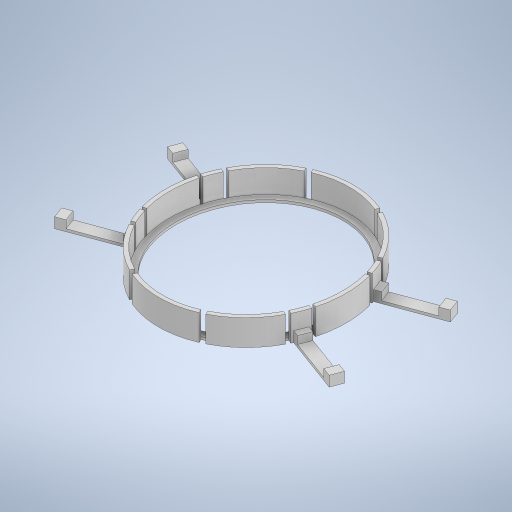
# Autodesk Inventor part: calibracao(0,5cm)
Saved by Autodesk Inventor 2024.3 (Build 283343000, 343)
## iProperties
Created: 2024-12-11
Part Number: calibracao(0,5cm)
Material: Genérico
Document SubType Name: Modeling
Designer: lostv
Density: 1 g/cm^3
Appearance: Padrão
Author: lostv
Autodesk Inventor part; units mm, degrees
ref_plane "YZ Plane" through (0, 0, 0) normal (1, 0, 0) x (0, 1, 0)
ref_plane "XZ Plane" through (0, 0, 0) normal (0, 1, 0) x (-1, 0, 0)
ref_plane "XY Plane" through (0, 0, 0) normal (0, 0, 1) x (1, 0, 0)
sketch "Esboço1" plane through (0, 0, 0) normal (0, 1, 0) x (-1, 0, 0)
  ellipse E0 centre (-16.8231, 43.9447) end of major axis (58.1769, 43.9447) minor radius 80.5 (58.1769, 43.9447) -> (-16.8231, 124.4447) ccw
  line L0 (-16.8231, 124.4447) -> (-16.8231, 43.9447) construction
  line L1 (-16.8231, 43.9447) -> (58.1769, 43.9447)
  line L2 (-16.8231, 43.9447) -> (38.0514, 98.8191) construction
  line L3 (-16.8231, 43.9447) -> (60.7811, 43.9447) construction
  line L4 (58.1769, 43.9447) -> (61.1769, 43.9447)
  ellipse E1 centre (-16.8231, 43.9447) end of major axis (-16.8231, 127.4447) minor radius 78 (36.942, 104.4388) -> (-11.8231, 127.273) ccw
  ellipse E2 centre (-16.8231, 43.9447) end of major axis (-16.8231, 127.4447) minor radius 78 (61.0369, 48.9447) -> (43.4965, 96.8842) ccw
  ellipse E3 centre (-16.8231, 43.9447) end of major axis (-16.8231, 127.4447) minor radius 78 (-21.8231, 127.273) -> (-70.5882, 104.4388) ccw
  ellipse E4 centre (-16.8231, 43.9447) end of major axis (-91.8231, 43.9447) minor radius 80.5 (-16.8231, 124.4447) -> (-91.8231, 43.9447) ccw
  line L5 (-16.8231, 43.9447) -> (-71.6976, 98.8191) construction
  line L6 (-16.8231, 43.9447) -> (-91.8231, 43.9447) construction
  line L7 (-16.8231, 43.9447) -> (-91.8231, 43.9447)
  ellipse E5 centre (-16.8231, 43.9447) end of major axis (-16.8231, 127.4447) minor radius 78 (-77.1427, 96.8842) -> (-94.6831, 48.9447) ccw
  line L8 (-96.047, 46.9447) -> (-91.771, 46.9447)
  line L9 (58.1769, 43.9447) -> (-91.8231, 43.9447)
  line L10 (-16.8231, 43.9447) -> (38.0514, -10.9298) construction
  ellipse E6 centre (-16.8231, 43.9447) end of major axis (58.1769, 43.9447) minor radius 80.5 (-16.8231, -36.5553) -> (58.1769, 43.9447) ccw
  line L11 (-16.8231, -36.5553) -> (-16.8231, 43.9447) construction
  line L12 (-13.8231, -40.7731) -> (-13.8231, -36.4909)
  line L13 (-11.8231, -40.7731) -> (-11.8231, -36.3762)
  line L14 (-13.8231, -36.4909) -> (-13.8231, -40.7731)
  ellipse E7 centre (-16.8231, 43.9447) end of major axis (-16.8231, -39.5553) minor radius 78 (-11.8231, -39.3836) -> (36.942, -16.5494) ccw
  ellipse E8 centre (-16.8231, 43.9447) end of major axis (-16.8231, -39.5553) minor radius 78 (43.4965, -8.9948) -> (61.0369, 38.9447) ccw
  line L15 (-69.7437, -13.0978) -> (-72.9021, -15.9416)
  line L16 (-73.673, -8.5619) -> (-76.9169, -11.4827)
  line L17 (-73.673, -8.5619) -> (-76.9169, -11.4827)
  line L18 (-69.7437, -13.0978) -> (-72.9021, -15.9416)
  line L19 (-19.8231, -40.7731) -> (-19.8231, -36.4909)
  line L20 (-19.8231, -36.4909) -> (-19.8231, -40.7731)
  line L21 (-21.8231, -40.7731) -> (-21.8231, -36.3762)
  ellipse E9 centre (-16.8231, 43.9447) end of major axis (-16.8231, -39.5553) minor radius 78 (-70.5882, -16.5494) -> (-21.8231, -39.3836) ccw
  line L22 (-16.8231, 43.9447) -> (-71.6976, -10.9298) construction
  ellipse E10 centre (-16.8231, 43.9447) end of major axis (-91.8231, 43.9447) minor radius 80.5 (-91.8231, 43.9447) -> (-16.8231, -36.5553) ccw
  ellipse E11 centre (-16.8231, 43.9447) end of major axis (-16.8231, -39.5553) minor radius 78 (-94.6831, 38.9447) -> (-77.1427, -8.9948) ccw
  line L23 (-96.047, 40.9447) -> (-91.8, 40.9447)
  line L24 (23.1769, -78.0731) -> (-56.8231, -78.0731)
  line L25 (-56.8231, -78.0731) -> (-56.8231, -78.0731)
  line L26 (-16.8231, -78.0731) -> (-16.8231, -84.5751) construction
  line L27 (-96.047, 38.9447) -> (-91.6783, 38.9447)
  line L28 (-96.047, 48.9447) -> (-91.6783, 48.9447)
  line L29 (-96.047, 38.9447) -> (-98.347, 38.9447) construction
  line L30 (-98.347, 38.9447) -> (-98.347, 41.4447) construction
  line L31 (-98.347, 41.4447) -> (-96.047, 41.4447) construction
  line L32 (-96.047, 38.9447) -> (-98.347, 38.9447)
  line L33 (-98.347, 41.4447) -> (-98.347, 38.9447)
  line L34 (-98.347, 41.4447) -> (-96.047, 41.4447)
  line L35 (-96.047, 41.4447) -> (-96.047, 40.9447)
  line L36 (-96.047, 46.9447) -> (-96.047, 46.4447)
  line L37 (-98.347, 46.4447) -> (-96.047, 46.4447)
  line L38 (-98.347, 46.4447) -> (-98.347, 48.9447)
  line L39 (-98.347, 48.9447) -> (-96.047, 48.9447)
  line L40 (-96.047, 40.9447) -> (-96.047, 41.4447) construction
  line L41 (-96.047, 46.4447) -> (-96.047, 46.9447) construction
  line L42 (-96.047, 41.4447) -> (-96.047, 46.4447)
  line L43 (-72.9021, -15.9416) -> (-76.9169, -11.4827) construction
  line L44 (-78.2551, -9.9964) -> (-74.9072, -6.9819)
  line L45 (-71.5638, -17.4279) -> (-68.3579, -14.5413)
  line L46 (-71.5638, -17.4279) -> (-73.2731, -18.9669)
  line L47 (-73.2731, -18.9669) -> (-74.9459, -17.109)
  line L48 (-74.9459, -17.109) -> (-73.2367, -15.57)
  line L49 (-72.9021, -15.9416) -> (-73.2367, -15.57)
  line L50 (-76.9169, -11.4827) -> (-73.2367, -15.57)
  line L51 (-78.2551, -9.9964) -> (-79.9644, -11.5354)
  line L52 (-79.9644, -11.5354) -> (-78.2915, -13.3933)
  line L53 (-78.2915, -13.3933) -> (-76.5823, -11.8543)
  line L54 (-13.8231, -40.7731) -> (-19.8231, -40.7731) construction
  line L55 (-21.8231, -40.7731) -> (-21.8231, -43.0731)
  line L56 (-21.8231, -43.0731) -> (-19.3231, -43.0731)
  line L57 (-19.3231, -43.0731) -> (-19.3231, -40.7731)
  line L58 (-19.8231, -40.7731) -> (-19.3231, -40.7731)
  line L59 (-11.8231, -40.7731) -> (-11.8231, -43.0731)
  line L60 (-11.8231, -43.0731) -> (-14.3231, -43.0731)
  line L61 (-14.3231, -43.0731) -> (-14.3231, -40.7731)
  line L62 (-13.8231, -40.7731) -> (-14.3231, -40.7731)
  line L63 (-19.3231, -40.7731) -> (-14.3231, -40.7731)
  line L64 (46.3182, -11.5354) -> (44.6453, -13.3933)
  line L65 (44.6089, -9.9964) -> (46.3182, -11.5354)
  line L66 (44.6453, -13.3933) -> (42.9361, -11.8543)
  line L67 (40.0268, -8.5619) -> (43.2707, -11.4827)
  line L68 (44.6089, -9.9964) -> (41.261, -6.9819)
  line L69 (43.2707, -11.4827) -> (39.5905, -15.57)
  line L70 (39.2559, -15.9416) -> (43.2707, -11.4827) construction
  line L71 (36.0975, -13.0978) -> (39.2559, -15.9416)
  line L72 (39.2559, -15.9416) -> (39.5905, -15.57)
  line L73 (41.2997, -17.109) -> (39.5905, -15.57)
  line L74 (39.6269, -18.9669) -> (41.2997, -17.109)
  line L75 (37.9176, -17.4279) -> (39.6269, -18.9669)
  line L76 (37.9176, -17.4279) -> (34.7117, -14.5413)
  line L77 (62.4009, 38.9447) -> (64.7009, 38.9447)
  line L78 (64.7009, 38.9447) -> (64.7009, 41.4447)
  line L79 (64.7009, 41.4447) -> (62.4009, 41.4447)
  line L80 (62.4009, 41.4447) -> (62.4009, 40.9447)
  line L81 (62.4009, 40.9447) -> (58.1538, 40.9447)
  line L82 (62.4009, 38.9447) -> (58.0321, 38.9447)
  line L83 (62.4009, 41.4447) -> (62.4009, 46.4447)
  line L84 (64.7009, 46.4447) -> (62.4009, 46.4447)
  line L85 (62.4009, 46.9447) -> (62.4009, 46.4447)
  line L86 (64.7009, 46.4447) -> (64.7009, 48.9447)
  line L87 (64.7009, 48.9447) -> (62.4009, 48.9447)
  line L88 (62.4009, 48.9447) -> (58.0321, 48.9447)
  line L89 (62.4009, 46.9447) -> (58.1248, 46.9447)
  line L90 (39.2559, 103.831) -> (39.5905, 103.4594)
  line L91 (37.9176, 105.3172) -> (39.6269, 106.8562)
  line L92 (39.6269, 106.8562) -> (41.2997, 104.9984)
  line L93 (41.2997, 104.9984) -> (39.5905, 103.4594)
  line L94 (39.2559, 103.831) -> (43.2707, 99.3721) construction
  line L95 (43.2707, 99.3721) -> (39.5905, 103.4594)
  line L96 (44.6453, 101.2827) -> (42.9361, 99.7437)
  line L97 (46.3182, 99.4248) -> (44.6453, 101.2827)
  line L98 (44.6089, 97.8858) -> (46.3182, 99.4248)
  line L99 (44.6089, 97.8858) -> (41.261, 94.8713)
  line L100 (40.0268, 96.4513) -> (43.2707, 99.3721)
  line L101 (36.0975, 100.9871) -> (39.2559, 103.831)
  line L102 (37.9176, 105.3172) -> (34.7117, 102.4306)
  line L103 (-71.5638, 105.3172) -> (-68.3579, 102.4306)
  line L104 (-71.5638, 105.3172) -> (-73.2731, 106.8562)
  line L105 (-73.2731, 106.8562) -> (-74.9459, 104.9984)
  line L106 (-74.9459, 104.9984) -> (-73.2367, 103.4594)
  line L107 (-72.9021, 103.831) -> (-73.2367, 103.4594)
  line L108 (-69.7437, 100.9871) -> (-72.9021, 103.831)
  line L109 (-76.9169, 99.3721) -> (-73.2367, 103.4594)
  line L110 (-78.2915, 101.2827) -> (-76.5823, 99.7437)
  line L111 (-73.673, 96.4513) -> (-76.9169, 99.3721)
  line L112 (-79.9644, 99.4248) -> (-78.2915, 101.2827)
  line L113 (-78.2551, 97.8858) -> (-79.9644, 99.4248)
  line L114 (-78.2551, 97.8858) -> (-74.9072, 94.8713)
  line L115 (-21.8231, 128.6625) -> (-21.8231, 130.9625)
  line L116 (-21.8231, 128.6625) -> (-21.8231, 124.2656)
  line L117 (-21.8231, 130.9625) -> (-19.3231, 130.9625)
  line L118 (-19.3231, 130.9625) -> (-19.3231, 128.6625)
  line L119 (-19.8231, 128.6625) -> (-19.3231, 128.6625)
  line L120 (-19.8231, 128.6625) -> (-19.8231, 124.3803)
  line L121 (-19.3231, 128.6625) -> (-14.3231, 128.6625)
  line L122 (-14.3231, 130.9625) -> (-14.3231, 128.6625)
  line L123 (-11.8231, 130.9625) -> (-14.3231, 130.9625)
  line L124 (-11.8231, 128.6625) -> (-11.8231, 124.2656)
  line L125 (-11.8231, 128.6625) -> (-11.8231, 130.9625)
  line L126 (-13.8231, 128.6625) -> (-13.8231, 124.3803)
  line L127 (-13.8231, 128.6625) -> (-19.8231, 128.6625) construction
  line L128 (-13.8231, 128.6625) -> (-14.3231, 128.6625)
  line L129 (58.1538, 40.9447) -> (58.1248, 40.9447)
  line L130 (-91.8, 40.9447) -> (-91.771, 40.9447)
  line L131 (-56.8231, -78.0731) -> (23.1769, -78.0731)
  line L132 (23.1769, -78.0731) -> (23.1769, -43.0731)
  line L133 (-56.8231, -43.0731) -> (-56.8231, -78.0731)
  line L134 (-16.8231, 43.9447) -> (-16.8231, 155.9447) construction
  line L135 (-16.8231, 43.9447) -> (89.6769, 43.9447) construction
  line L136 (-16.8231, 43.9447) -> (-16.8231, -64.5553) construction
  line L137 (-16.8231, 43.9447) -> (-123.3231, 43.9447) construction
  line L138 (-16.8231, 43.9447) -> (92.6769, 43.9447) construction
  line L139 (-16.8231, 43.9447) -> (-126.3231, 43.9447) construction
  line L140 (-16.8231, 43.9447) -> (-16.8231, 158.9447) construction
  line L141 (-16.8231, 43.9447) -> (-16.8231, -67.5553) construction
  line L142 (-14.3231, -43.0731) -> (-14.3231, -40.7731)
  line L143 (-19.3231, -40.7731) -> (-19.3231, -43.0731)
  line L144 (-19.3231, -40.7731) -> (-14.3231, -40.7731)
  line L145 (23.1769, -43.0731) -> (-14.3231, -43.0731)
  line L146 (-19.3231, -43.0731) -> (-56.8231, -43.0731)
  ellipse E12 centre (-16.8231, 43.9447) end of major axis (92.6769, 43.9447) minor radius 115 (23.1769, -63.1078) -> (-56.8231, -63.1078) ccw
  line L147 (81.5648, 71.8126) -> (78.4536, 83.201)
  line L148 (78.4536, 83.201) -> (82.5191, 84.3116)
  line L149 (81.5648, 71.8126) -> (86.023, 73.0305)
  line L150 (-115.211, 71.8126) -> (-119.6692, 73.0305)
  line L151 (-115.211, 71.8126) -> (-112.0998, 83.201)
  line L152 (-112.0998, 83.201) -> (-116.1653, 84.3116)
  ellipse E13 centre (-16.8231, 43.9447) end of major axis (89.6769, 43.9447) minor radius 112 (23.1769, -59.8555) -> (86.023, 73.0305) ccw
  ellipse E14 centre (-16.8231, 43.9447) end of major axis (89.6769, 43.9447) minor radius 112 (82.5191, 84.3116) -> (-116.1653, 84.3116) ccw
  ellipse E15 centre (-16.8231, 43.9447) end of major axis (89.6769, 43.9447) minor radius 112 (-119.6692, 73.0305) -> (-56.8231, -59.8555) ccw
  circle A0 centre (16.1769, -50.0731) radius 1.75
  circle A1 centre (-49.8231, -50.0731) radius 1.75
  line L153 (89.5899, 93.6335) -> (44.298, 76.9085)
  line L154 (44.298, 76.9085) -> (47.1282, 68.1314)
  line L155 (47.1282, 68.1314) -> (92.7817, 84.99)
  line L156 (92.7817, 84.99) -> (89.5899, 93.6335)
  line L157 (89.5899, -5.7442) -> (44.298, 10.9809)
  line L158 (44.298, 10.9809) -> (47.1282, 19.758)
  line L159 (47.1282, 19.758) -> (92.7817, 2.8994)
  line L160 (92.7817, 2.8994) -> (89.5899, -5.7442)
  line L161 (-123.2361, 93.6335) -> (-77.9442, 76.9085)
  line L162 (-77.9442, 76.9085) -> (-80.7744, 68.1314)
  line L163 (-80.7744, 68.1314) -> (-126.4279, 84.99)
  line L164 (-126.4279, 84.99) -> (-123.2361, 93.6335)
  line L165 (-123.2361, -5.7442) -> (-77.9442, 10.9809)
  line L166 (-80.7744, 19.758) -> (-126.4279, 2.8994)
  line L167 (-126.4279, 2.8994) -> (-123.2361, -5.7442)
  line L168 (-77.9442, 10.9809) -> (-80.7744, 19.758)
  line L169 (-16.8231, 43.9447) -> (-16.8231, -31.5553) construction
  line L170 (-16.8231, 43.9447) -> (53.1769, 43.9447) construction
  ellipse E16 centre (-16.8231, 43.9447) end of major axis (-16.8231, -31.5553) minor radius 70
  line L171 (-16.8231, 43.9447) -> (-16.8231, -28.5553) construction
  line L172 (-16.8231, 43.9447) -> (50.1769, 43.9447) construction
  ellipse E17 centre (-16.8231, 43.9447) end of major axis (-16.8231, -28.5553) minor radius 67
  line L173 (9.1801, 114.0421) -> (7.9104, 111.3238)
  line L174 (12.7897, 112.3561) -> (11.5281, 109.634)
  line L175 (9.1801, -26.1528) -> (7.9104, -23.4345)
  line L176 (12.7897, -24.4667) -> (11.5281, -21.7446)
  line L177 (-42.8263, 114.0421) -> (-41.5566, 111.3238)
  line L178 (-46.4359, 112.3561) -> (-45.1743, 109.634)
  line L179 (-42.8263, -26.1528) -> (-41.5566, -23.4345)
  line L180 (-46.4359, -24.4667) -> (-45.1743, -21.7446)
  line L181 (-77.4369, 81.7095) -> (-74.7161, 80.4386)
  line L182 (-76.0765, 77.7854) -> (-78.8404, 78.9584)
  line L183 (-80.4928, 66.5177) -> (-83.3871, 67.3084)
  line L184 (-81.1396, 64.2577) -> (-84.0231, 65.0848)
  line L185 (43.7907, 81.7095) -> (41.0699, 80.4386)
  line L186 (42.4303, 77.7854) -> (45.1942, 78.9584)
  line L187 (46.8466, 66.5177) -> (49.7409, 67.3084)
  line L188 (47.4934, 64.2577) -> (50.3769, 65.0848)
  line L189 (-77.4369, 6.1798) -> (-74.7161, 7.4508)
  line L190 (-76.0765, 10.1039) -> (-78.8404, 8.931)
  line L191 (-80.4928, 21.3717) -> (-83.3871, 20.581)
  line L192 (-81.1396, 23.6316) -> (-84.0231, 22.8046)
  line L193 (47.4934, 23.6316) -> (50.3769, 22.8046)
  line L194 (46.8466, 21.3717) -> (49.7409, 20.581)
  line L195 (42.4303, 10.1039) -> (45.1942, 8.931)
  line L196 (43.7907, 6.1798) -> (41.0699, 7.4508)
  line L197 (-16.8231, 43.9447) -> (45.1769, 43.9447)
  line L198 (-16.8231, 43.9447) -> (-16.8231, -23.5553)
  ellipse E18 centre (-16.8231, 43.9447) end of major axis (45.1769, 43.9447) minor radius 67.5
  point P0 (0, 0)
  point P1 (78.1769, 43.9447)
  point P2 (81.1769, 43.9447)
  point P3 (-100.7855, 43.9447)
  point P4 (-72.3567, -15.4505)
  point P5 (-97.197, 41.4447)
  point P6 (-97.197, 38.9447)
  point P7 (-96.047, 41.1947)
  point P8 (-96.047, 46.6947)
  point P9 (-97.197, 48.9447)
  point P10 (-93.8627, 48.9447)
  point P11 (-72.4185, -18.1974)
  point P12 (-77.4369, -12.6238)
  point P13 (-79.128, -12.4643)
  point P14 (-14.3231, -41.9231)
  point P15 (-19.5731, -40.7731)
  point P16 (-13.8231, -38.632)
  point P17 (62.4009, 41.1947)
  point P18 (-96.047, 43.9447)
  point P19 (-58.2564, -59.4853)
  point P20 (24.6102, -59.4853)
  point P21 (23.1769, -57.0582)
  point P22 (-13.0731, 130.9625)
  point P23 (64.7009, 40.1947)
  point P24 (-82.8852, 68.9108)
  point P25 (-79.532, 77.4948)
  point P26 (-84.2338, 79.231)
  point P27 (-87.5779, 70.6437)
  point P28 (-79.532, 10.3946)
  point P29 (-82.8852, 18.9785)
  point P30 (-87.5779, 17.2456)
  point P31 (-84.2338, 8.6583)
  point P32 (-119.9522, 82.5987)
  point P33 (-116.6506, 91.2017)
  point P34 (-116.6506, -3.3123)
  point P35 (-119.9522, 5.2907)
  point P36 (83.0044, 91.2017)
  point P37 (86.306, 82.5987)
  point P38 (45.8858, 77.4948)
  point P39 (49.239, 68.9108)
  point P40 (53.9317, 70.6437)
  point P41 (50.5876, 79.231)
  point P42 (86.306, 5.2907)
  point P43 (83.0044, -3.3123)
  point P44 (49.239, 18.9785)
  point P45 (45.8858, 10.3946)
  point P46 (50.5876, 8.6583)
  point P47 (53.9317, 17.2456)
  dimension "d3" = 83.5
  dimension "d4" = 78
  dimension "d0" = 75
  dimension "d1" = 80.5
  dimension "d2" = 45
  dimension "d5" = 2.5
  dimension "d6" = 2
  dimension "d7" = 2.3
  dimension "d8" = 2.3
  dimension "d9" = 2
  dimension "d10" = 2.5
  dimension "d11" = 6.6688
  dimension "d12" = 2.5
  dimension "d13" = 2.5
  dimension "d14" = 2.3
  dimension "d15" = 2.5
  dimension "d16" = 2.5
  dimension "d17" = 2.3
  dimension "d18" = 4.2822
  dimension "d19" = 6
  dimension "d20" = 112
  dimension "d21" = 106.5
  dimension "d22" = 106.5
  dimension "d23" = 109.5
  dimension "d24" = 109.5
  dimension "d25" = 115
  dimension "d26" = 24.9822
  dimension "d27" = 24.9761
  dimension "d28" = 80
  dimension "d29" = 40
  dimension "d30" = 35
  dimension "d31" = 3.5
  dimension "d32" = 7
  dimension "d33" = 7
  dimension "d34" = 75.5
  dimension "d35" = 70
  dimension "d36" = 72.5
  dimension "d37" = 67
  dimension "d46" = 62
  dimension "d47" = 67.5
  constraints: 398 end point, 148 symmetric about line, 55 point on line, 22 perpendicular, 18 coincident, 18 horizontal, 16 midpoint, 14 vertical, 12 collinear, 5 parallel, 2 centre point, 1 equal length, 129 other
  measures "d0" distance of L1.start L1.end
  measures "d1" distance of L0.start L1.start
  measures "d2" angle of L3 L2
  measures "d5" distance of point (-97.197, 41.445) point (-97.197, 38.945)
  measures "d6" distance between parallel lines of L27 L23
  measures "d7" distance from line of point (-96.047, 41.195) L33
  measures "d8" distance from line of point (-96.047, 46.695) L38
  measures "d9" distance from line of L8 point (-93.863, 48.945)
  measures "d10" distance from line of point (-97.197, 48.945) L37
  measures "d11" distance of L27.end L29.end
  measures "d12" distance from line of point (-72.418, -18.197) L48
  measures "d13" distance from line of point (-77.437, -12.624) L51
  measures "d14" distance between parallel lines of L43 L52
  measures "d15" distance between parallel lines of L57 L55
  measures "d16" distance from line of L59 point (-14.323, -41.923)
  measures "d17" distance from line of point (-19.573, -40.773) L56
  measures "d18" distance of L58.start L20.start
  measures "d19" distance from line of point (-13.823, -38.632) L19
  measures "d20" distance of L135.start L134.end
  measures "d21" distance of L135.start L135.end
  measures "d22" distance of L135.start L137.end
  measures "d23" distance of L138.start L138.end
  measures "d24" distance of L138.start L139.end
  measures "d25" distance of L138.start L140.end
  measures "d26" vertical distance of point (-13.073, 130.962) L134.end
  measures "d27" horizontal distance of point (64.701, 40.195) L135.end
  measures "d28" distance between parallel lines of L132 L133
  measures "d29" distance between parallel lines of L136 L132
  measures "d30" distance of L133.start L25.end
  measures "d31" diameter of A0
  measures "d32" distance from line of L132 A0.centre
  measures "d33" distance from line of L145 A0.centre
  measures "d34" distance of L169.start L169.end
  measures "d35" distance of L169.start L170.end
  measures "d36" distance of L171.start L171.end
  measures "d37" distance of L171.start L172.end
  measures "d46" distance of L197.start L197.end
  measures "d47" distance of L198.start L198.end
extrude "Extrusão1" add sketch "Esboço1" along normal blind 2 contours E17 L7 E18 L1 | L1 E18 L7 E17
extrude "Extrusão2" add sketch "Esboço1" along normal blind 20 contours E16 L193 E17 L1 | L1 E17 L188 E16 | E16 L159 L158 L157 L195 E17 L194 | L187 E17 L186 E16 L153 L154 L155 | L155 L154 L153 E16 | E16 L157 L158 L159 | E17 L192 E16 L7 | L7 E16 L184 E17 | L196 E16 L176 E17 | E17 L174 E16 L185 | L183 E16 L163 L162 L161 L182 E17 | E17 L190 E16 L165 L168 L166 L191 | L175 E16 L179 E17 | E17 L177 E16 L173 | L161 L162 L163 E16 | L166 L168 L165 E16 | L181 E16 L178 E17 | E17 L180 E16 L189
extrude "Extrusão3" add sketch "Esboço1" along normal blind 8 contours L155 E16 L153 E0 | E6 L157 E16 L159 | E12 L153 L156 L155 | L159 L160 L157 E12 | E12 L163 L164 L161 | L161 E16 L163 E4 | E12 L165 L167 L166 | E16 L165 E10 L166
extrude "Extrusão4" add sketch "Esboço1" along normal blind 2 contours E0 L153 E2 L155 | L159 E8 L157 E6 | E2 L153 E14 L148 L147 L155 | L159 E13 L157 E8 | L147 L148 E14 L153 E12 L155 | L159 E12 L157 E13 | L161 E5 L163 L151 L152 E14 | E14 L152 L151 L163 E12 L161 | L161 E4 L163 E5 | L166 E15 L165 E12 | L166 E11 L165 E15 | E10 L165 E11 L166
